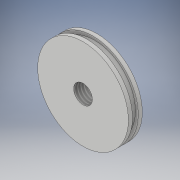
# Autodesk Inventor part: piston_deplaceur
Saved by Autodesk Inventor 2019 (Build 230136000, 136)
## iProperties
Created: 2019-03-19
Part Number: piston_deplaceur
Material: Générique
Document SubType Name: Modeling
Designer: theor
Density: 1 g/cm^3
Appearance: Par défaut
Author: theor
Autodesk Inventor part; units mm, degrees
ref_plane "YZ Plane" through (0, 0, 0) normal (1, 0, 0) x (0, 1, 0)
ref_plane "XZ Plane" through (0, 0, 0) normal (0, 1, 0) x (-1, 0, 0)
ref_plane "XY Plane" through (0, 0, 0) normal (0, 0, 1) x (1, 0, 0)
sketch "Esquisse2" plane through (0, 0, 0) normal (1, 0, 0) x (0, 1, 0)
  line L0 (0, 0) -> (0, -10.0642)
  line L1 (7.25, 2.2281) -> (7.25, 1.5734)
  line L2 (7.25, 1.5734) -> (6.55, 1.8281)
  line L3 (6.55, 1.8281) -> (6.55, 0.4)
  line L4 (6.55, 0.4) -> (7.25, 0.6548)
  line L5 (7.25, 0.6548) -> (7.25, 0)
  circle A0 centre (7.05, 1.1141) radius 0.5 construction
  line L6 (7.25, 2.2281) -> (1.5, 2.2281)
  line L7 (7.25, 0) -> (1.5, 0)
  line L8 (1.5, 0) -> (1.5, 2.2281)
  dimension "d1" = 1
  dimension "d2" = 70
  dimension "d3" = 70
  dimension "d4" = 0.2
  dimension "d5" = 14.5
  dimension "d7" = 0.4
  dimension "d8" = 0.4
  dimension "d9" = 3
  constraints: 18 end point, 4 vertical, 3 tangent, 2 horizontal, 2 point on line, 1 centre point, 1 horizontal alignment
  measures "d1" diameter of A0
  measures "d2" angle of L4 L3
  measures "d3" angle of L2 L3
  measures "d4" distance from line of L1 A0.centre
  measures "d5" diameter of L5 L0
  measures "d7" vertical distance of L5.end L3.end
  measures "d8" vertical distance of L1.start L2.end
  measures "d9" diameter of L8 L0
revolve "Révolution1" add sketch "Esquisse2" angle 360 about axis through (0, 0, 0) along (0, 0, -1)
thread "Filetage1" size "M3x0.5" class "6H" standard "ISO Metric profile" full length
equation "\"d3\" = d2"
equation "\"d8\" = d7"
